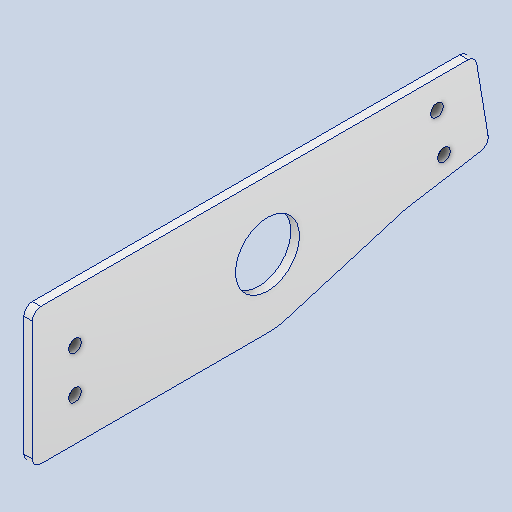
# Autodesk Inventor part: dribl-v3-Plate-2
Saved by Autodesk Inventor 2025.2 (Build 292293000, 293)
## iProperties
Created: 2025-04-04
Part Number: dribl-v3-Plate-2
Material: アルミニウム 6061
Document SubType Name: Modeling
Designer: haruy
Density: 2.7 g/cm^3
Appearance: アルミニウム - フラット
Author: haruy
Autodesk Inventor part; units mm, degrees
ref_plane "YZ Plane" through (0, 0, 0) normal (1, 0, 0) x (0, 1, 0)
ref_plane "XZ Plane" through (0, 0, 0) normal (0, 1, 0) x (-1, 0, 0)
ref_plane "XY Plane" through (0, 0, 0) normal (0, 0, 1) x (1, 0, 0)
derived "dribl-v3-Sketch-Base.ipt"
sketch "スケッチ1" plane through (400, 0, 0) normal (1, 0, 0) x (0, 1, 0)
  circle A0 centre (0, 0) radius 120 construction
  circle A1 centre (-96.5237, 35.1318) radius 6.5
  line L0 (0, 0) -> (-96.5237, 35.1318)
  line L1 (0, 0) -> (0, 120)
  line L2 (246.0862, 200) -> (-251.4603, 200)
  circle A2 centre (-67.6203, 200) radius 6.5
  line L3 (0, 0) -> (-120, 0)
  line L4 (248, 9.15) -> (186, 9.15)
  line L5 (186, 9.15) -> (186, -9.15)
  line L6 (186, -9.15) -> (248, -9.15)
  line L7 (248, -9.15) -> (248, 9.15)
  line L8 (186, 5.15) -> (178, 5.15)
  line L9 (178, 5.15) -> (178, -4.85)
  line L10 (178, -4.85) -> (186, -4.85)
  line L11 (186, -4.85) -> (186, 5.15)
  line L12 (178, 3.15) -> (173, 3.15)
  line L13 (173, 3.15) -> (173, -2.85)
  line L14 (173, -2.85) -> (178, -2.85)
  line L15 (178, -2.85) -> (178, 3.15)
  line L16 (173, 2.65) -> (158, 2.65)
  line L17 (158, 2.65) -> (158, -2.35)
  line L18 (158, -2.35) -> (173, -2.35)
  line L19 (173, -2.35) -> (173, 2.65)
  line L20 (186, 34.15) -> (184, 34.15)
  line L21 (184, 34.15) -> (184, -47.85)
  line L22 (184, -47.85) -> (186, -47.85)
  line L23 (186, -47.85) -> (186, 34.15)
  circle A3 centre (150, 65) radius 4
  circle A4 centre (150, 65) radius 14 construction
  line L24 (186, 34.15) -> (191, 34.15)
  line L25 (191, 34.15) -> (191, 14.15)
  line L26 (191, 14.15) -> (186, 14.15)
  line L27 (186, 14.15) -> (186, 34.15)
  line L28 (184, 34.15) -> (147.5804, 61.8148)
  line L29 (151.3835, 68.7531) -> (191, 54.15)
  line L30 (191, 54.15) -> (191, 34.15)
  line L31 (239.3868, 130) -> (-239.3868, 130)
  circle A5 centre (-96.5237, 35.1318) radius 4
  circle A6 centre (150, 65) radius 9
  line L32 (-92.7649, 33.7637) -> (-100.2825, 36.4998)
  line L33 (165, 36) -> (150, 36)
  circle A7 centre (150, 36) radius 5
  circle A8 centre (150, 36) radius 9
  circle A9 centre (-98.8174, 128.095) radius 6.5
  circle A10 centre (165, 36) radius 5
  line L34 (150, 65) -> (165, 36)
  circle A11 centre (165, 36) radius 9
  circle A12 centre (150, 65) radius 41.6497
  line L35 (150, 65) -> (150, 36)
  line L36 (150, 65) -> (-96.5237, 35.1318)
  line L37 (-98.8174, 128.095) -> (150, 65)
  line L38 (150, 65) -> (150, 23.3503)
  circle A13 centre (150, 65) radius 32.6497
  circle A14 centre (150, 32.3503) radius 9
  line L39 (166.9362, 23.3503) -> (134.8586, 23.3503)
  line L40 (174, 3.15) -> (174, -2.85)
  circle A15 centre (25, 0) radius 120
  line L41 (170, -52.2973) -> (211.3465, -67.3462)
  line L42 (211.3465, -67.3462) -> (205.1901, -84.2607)
  line L43 (205.1901, -84.2607) -> (163.8436, -69.2118)
  line L44 (163.8436, -69.2118) -> (170, -52.2973)
  line L45 (166.9218, -60.7546) -> (0, 0)
  line L46 (172.8191, -53.3234) -> (166.6627, -70.2379)
  line L47 (186, -47.85) -> (172.8191, -53.3234)
  line L48 (182.216, -56.7436) -> (176.0596, -73.6581)
  line L49 (186, -47.85) -> (191, -47.85)
  line L50 (191, -47.85) -> (191, -37.85)
  line L51 (191, -37.85) -> (186, -37.85)
  line L52 (186, -37.85) -> (186, -47.85)
  line L53 (191, -47.85) -> (182.216, -56.7436)
  circle A16 centre (221.5, -275) radius 6
  line L54 (211.5, 20) -> (208.5, 20)
  line L55 (208.5, 20) -> (208.5, -53.7075)
  line L56 (208.5, -53.7075) -> (211.5, -53.7075)
  line L57 (211.5, -53.7075) -> (211.5, 20)
  line L58 (211.5, 20) -> (231.5, 20)
  line L59 (231.5, 20) -> (231.5, -53.7075)
  line L60 (231.5, -53.7075) -> (211.5, -53.7075)
  line L61 (211.5, -53.7075) -> (211.5, 20)
  line L62 (-432.3334, -230) -> (-447.3334, -230) construction
  line L63 (-447.3334, -230) -> (-447.3334, -860) construction
  line L64 (-447.3334, -860) -> (-432.3334, -860) construction
  line L65 (-432.3334, -860) -> (-432.3334, -230) construction
  line L66 (-432.3334, -250) -> (-432.3334, -230) construction
  line L67 (343, -291.5) -> (278.5, -291.5)
  line L68 (278.5, -291.5) -> (278.5, -334.5)
  line L69 (278.5, -334.5) -> (343, -334.5)
  line L70 (343, -334.5) -> (343, -291.5)
  line L71 (278.5, -291.5) -> (293.5, -291.5)
  line L72 (293.5, -291.5) -> (293.5, -276.5)
  line L73 (293.5, -276.5) -> (278.5, -276.5)
  line L74 (278.5, -276.5) -> (278.5, -291.5)
  line L75 (211.5, -53.7075) -> (231.5, -53.7075)
  line L76 (231.5, -53.7075) -> (231.5, -305)
  line L77 (231.5, -305) -> (211.5, -305)
  line L78 (211.5, -305) -> (211.5, -53.7075)
  line L79 (-432.3334, -303) -> (-447.3334, -303)
  line L80 (-432.3334, -303) -> (875.6666, -303)
  line L81 (875.6666, -303) -> (875.6666, -323)
  line L82 (875.6666, -323) -> (-432.3334, -323)
  line L83 (-432.3334, -323) -> (-432.3334, -303)
  line L84 (278.5, -334.5) -> (293.5, -334.5)
  line L85 (293.5, -334.5) -> (293.5, -349.5)
  line L86 (293.5, -349.5) -> (278.5, -349.5)
  line L87 (278.5, -349.5) -> (278.5, -334.5)
  line L88 (278.5, -276.5) -> (263.5, -276.5)
  line L89 (263.5, -276.5) -> (263.5, -359.5)
  line L90 (263.5, -359.5) -> (278.5, -359.5)
  line L91 (278.5, -359.5) -> (278.5, -276.5)
  circle A17 centre (221.5, -275) radius 15
  line L92 (231.5, -275) -> (211.5, -275)
  line L93 (211.5, -275) -> (211.5, -305)
  line L94 (211.5, -305) -> (231.5, -305)
  line L95 (231.5, -305) -> (231.5, -275)
  line L96 (226.5, -266.3397) -> (216.5, -283.6603)
  line L97 (242.4808, -298.6603) -> (252.4808, -281.3397)
  line L98 (216.5, -283.6603) -> (242.4808, -298.6603)
  line L99 (-524.3334, 10.1879) -> (-524.3334, -1075.6286) construction
  line L100 (278.5, -349.5) -> (263.5, -349.5)
  line L101 (278.5, -276.5) -> (225.8253, -260.6372)
  line L102 (263.5, -349.5) -> (209.9279, -284.544)
  line L103 (278.5, -313) -> (263.5, -313)
  circle A18 centre (271, -291.5) radius 1.6
  circle A19 centre (271, -334.5) radius 1.6
  circle A20 centre (221.5, -275) radius 9.1
  circle A21 centre (221.5, -275) radius 50
  circle A22 centre (239.5, -334.8519) radius 12.5
  line L104 (221.5, -275) -> (237.3114, -322.4342)
  line L105 (221.5, -275) -> (178.1987, -300)
  line L106 (221.5, -275) -> (221.5, -225)
  line L107 (221.5, -275) -> (254.6735, -237.5899)
  circle A23 centre (259.5, -334.8519) radius 4
  circle A24 centre (239.5, -354.8519) radius 4
  circle A25 centre (219.5, -334.8519) radius 4
  line L108 (206.6714, -277.2613) -> (215.5457, -335.4549)
  line L109 (216.6716, -337.6803) -> (236.6716, -357.6803)
  line L110 (263.5, -349.5) -> (240.9941, -358.5624)
  circle A26 centre (259.5, -334.8519) radius 1.6
  circle A27 centre (239.5, -354.8519) radius 1.6
  circle A28 centre (219.5, -334.8519) radius 1.6
  line L111 (-452.3334, -283) -> (-432.3334, -283)
  line L112 (-432.3334, -283) -> (-432.3334, -663)
  line L113 (-432.3334, -663) -> (-452.3334, -663)
  line L114 (-452.3334, -663) -> (-452.3334, -283)
  line L115 (-464.8334, 407.9273) -> (-464.8334, -989.4099)
  line L116 (1035.1666, 407.9273) -> (1035.1666, -2194.3714)
  line L117 (-432.3334, -643) -> (-452.3334, -643)
  line L118 (-432.3334, -473) -> (-464.8334, -473)
  line L119 (-464.8334, -88) -> (1035.1666, -88)
  line L120 (1035.1666, 77) -> (-464.8334, 77)
  line L121 (875.6666, -303) -> (1005.1666, -303)
  line L122 (1005.1666, -303) -> (1005.1666, -323)
  line L123 (1005.1666, -323) -> (875.6666, -323)
  line L124 (875.6666, -323) -> (875.6666, -303)
  line L125 (1005.1666, -303) -> (980.1666, -303)
  line L126 (980.1666, -303) -> (980.1666, -323)
  line L127 (980.1666, -323) -> (1005.1666, -323)
  line L128 (1005.1666, -323) -> (1005.1666, -303)
  circle A29 centre (964.1666, -358.18) radius 16
  circle A30 centre (964.1666, -358.18) radius 7.5
  line L129 (976.8707, -387.2746) -> (-428.6466, -622.1068)
  line L130 (-428.6466, -622.1068) -> (-425.3507, -641.8333)
  line L131 (-425.3507, -641.8333) -> (980.1666, -407.0011)
  line L132 (980.1666, -407.0011) -> (976.8707, -387.2746)
  line L133 (-432.3334, -643) -> (-425.3507, -641.8333)
  line L134 (980.1666, -323) -> (980.1666, -407.0011)
  line L135 (-212.3334, -323) -> (-232.3334, -323)
  line L136 (-232.3334, -323) -> (-232.3334, -578)
  line L137 (-232.3334, -578) -> (-212.3334, -578)
  line L138 (-212.3334, -578) -> (-212.3334, -323)
  line L139 (-414.8334, 0) -> (-414.8334, -960.8427)
  line L140 (-432.3334, -323) -> (-432.3334, -622.7228)
  line L141 (-232.3334, 0) -> (-232.3334, -854.7037)
  line L142 (-232.3334, -303) -> (-127.3334, -303)
  line L143 (-127.3334, -303) -> (-127.3334, -379.18)
  line L144 (-127.3334, -379.18) -> (-232.3334, -379.18)
  line L145 (-232.3334, -379.18) -> (-232.3334, -303)
  line L146 (-164.3334, -303) -> (-184.3334, -303)
  line L147 (-184.3334, -303) -> (-184.3334, -323)
  line L148 (-184.3334, -323) -> (-164.3334, -323)
  line L149 (-164.3334, -323) -> (-164.3334, -303)
  line L150 (985.1666, -303) -> (985.1666, -323)
  circle A31 centre (-222.3334, -313) radius 1.6
  circle A32 centre (-202.3334, -313) radius 1.6
  circle A33 centre (-222.3334, -333) radius 1.6
  circle A34 centre (-222.3334, -353) radius 1.6
  circle A35 centre (-139.3334, -313) radius 1.6
  circle A36 centre (-149.3334, -313) radius 1.6
  circle A37 centre (-143.3334, -358.18) radius 16
  line L151 (948.1666, -303) -> (948.1666, -323)
  circle A38 centre (968.1666, -313) radius 1.5
  circle A39 centre (958.1666, -313) radius 1.5
  line L152 (957.1441, -390.5705) -> (960.44, -410.297)
  circle A40 centre (973.587, -397.9618) radius 1.5
  circle A41 centre (963.7237, -399.6098) radius 1.5
  line L153 (948.1666, -323) -> (948.1666, -358.18)
  line L154 (957.1441, -390.5705) -> (948.8361, -362.7598)
  circle A42 centre (-422.3334, -313) radius 1.6
  circle A43 centre (-412.3334, -313) radius 1.6
  circle A44 centre (-402.3334, -313) radius 1.6
  circle A45 centre (-417.1354, -630.3221) radius 1.6
  circle A46 centre (-407.2721, -628.6742) radius 1.6
  circle A47 centre (-442.3334, -633) radius 1.6
  circle A48 centre (-442.3334, -623) radius 1.6
  line L155 (-452.3334, -613) -> (-432.3334, -613)
  line L156 (-399.0568, -617.1629) -> (-395.7609, -636.8895)
  line L157 (-428.6466, -622.1068) -> (-432.3334, -622.7228)
  line L158 (-232.3334, -193) -> (-212.3334, -193)
  line L159 (-212.3334, -193) -> (-212.3334, -753)
  line L160 (-212.3334, -753) -> (-232.3334, -753)
  line L161 (-232.3334, -753) -> (-232.3334, -193)
  line L162 (-212.3334, -443) -> (-192.3334, -443)
  line L163 (-192.3334, -443) -> (-192.3334, -463)
  line L164 (-192.3334, -463) -> (-212.3334, -463)
  line L165 (-212.3334, -463) -> (-212.3334, -443)
  line L166 (-212.3334, -593) -> (-192.3334, -593)
  line L167 (-192.3334, -593) -> (-192.3334, -613)
  line L168 (-192.3334, -613) -> (-212.3334, -613)
  line L169 (-212.3334, -613) -> (-212.3334, -593)
  line L170 (-212.3334, -638) -> (162.6666, -638)
  line L171 (162.6666, -638) -> (162.6666, -653)
  line L172 (162.6666, -653) -> (-212.3334, -653)
  line L173 (-212.3334, -653) -> (-212.3334, -638)
  line L174 (162.6666, -653) -> (177.6666, -653)
  line L175 (177.6666, -653) -> (177.6666, -668)
  line L176 (177.6666, -668) -> (162.6666, -668)
  line L177 (162.6666, -668) -> (162.6666, -653)
  line L178 (162.6666, -668) -> (147.6666, -668)
  line L179 (147.6666, -668) -> (147.6666, -524.7026)
  line L180 (147.6666, -524.7026) -> (162.6666, -524.7026)
  line L181 (162.6666, -524.7026) -> (162.6666, -668)
  circle A49 centre (155.1666, -534.7026) radius 1.6
  circle A50 centre (835.5011, -421.0331) radius 1.6
  circle A51 centre (855.2277, -417.7372) radius 1.6
  point P0 (-60, 0)
  point P1 (875.6666, -313)
  point P2 (186, 0.15)
  point P3 (186, 0)
extrude "押し出し1" add sketch "スケッチ1" along normal blind 2 contours L154 A29 L134 L132 L129 | L129 L132 L131 L152 | A29 | L121 L126 L123 L151 | L153 L123 L134 A29
fillet "フィレット1" radius 2 4 edges at (401, 980.1666, -303) (401, 948.1666, -303) (401, 960.44, -410.297) (401, 980.1666, -407.0011)
